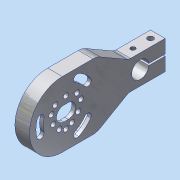
# Autodesk Inventor part: MotorMountingPlate
Saved by Autodesk Inventor 2015 SP1 (Build 190203100, 203)
## iProperties
Created: 2015-06-16
Part Number: MotorMountingPlate
Material: Aluminum 6061
Document SubType Name: Modeling
Designer: YOUR_NAME_HERE
Density: 2.7 g/cm^3
Appearance: Aluminum - Flat
Mass: 93.3221 g
Surface Area: 173.371 cm^2
Volume: 34.5637 cm^3
Author: YOUR_NAME_HERE
Autodesk Inventor part; units mm, degrees
ref_plane "YZ Plane" through (0, 0, 0) normal (1, 0, 0) x (0, 1, 0)
ref_plane "XZ Plane" through (0, 0, 0) normal (0, 1, 0) x (-1, 0, 0)
ref_plane "XY Plane" through (0, 0, 0) normal (0, 0, 1) x (1, 0, 0)
sketch "Sketch1" plane through (0, 0, 0) normal (1, 0, 0) x (0, 1, 0)
  circle A0 centre (0, 0) radius 31.85 construction
  circle A1 centre (0, 64.66) radius 12.75 construction
  line L0 (-44.59, 0) -> (44.59, 0) projected
  line L1 (0, -57.502) -> (0, 122.062) projected
  line L2 (28.575, 96.41) -> (-28.575, 96.41)
  line L3 (-28.575, 96.41) -> (-28.575, -21.59)
  line L4 (-28.575, -21.59) -> (28.575, -21.59)
  line L5 (28.575, -21.59) -> (28.575, 96.41)
  circle A2 centre (0, 64.66) radius 6.35
  circle A3 centre (0, 0) radius 7.5
  dimension "d0" = 63.7
  dimension "d1" = 25.5
  dimension "CC" = 64.66
  dimension "d3" = 21.59
  dimension "d4" = 28.575
  dimension "d5" = 31.75
  dimension "d6" = 15
  dimension "d7" = 12.7
  constraints: 8 end point, 4 centre point, 2 coincident, 2 parallel, 1 horizontal, 1 perpendicular, 1 point on line, 1 other
  measures "d0" diameter of A0
  measures "d1" diameter of A1
  measures "CC" distance of A0.centre A1.centre
  measures "d3" distance from line of L4 A0.centre
  measures "d4" distance from line of L5 A0.centre
  measures "d5" distance from line of A1.centre L2
  measures "d6" diameter of A3
  measures "d7" diameter of A2
extrude "Extrusion1" add sketch "Sketch1" along normal blind 12.7 contours L3 L2 L1 A2 A3 L0 | L0 A3 L1 L4 L3 | L1 A2 L2 L5 L0 A3 | A3 L0 L5 L4 L1
sketch "Sketch2" plane through (12.7, 0, 0) normal (1, 0, 0) x (0, 0, -1)
  circle A0 centre (-64.66, 0) radius 6.35 projected
  circle A1 centre (-64.66, 0) radius 12.5 construction
  circle A2 centre (-64.66, 12.5) radius 2.25
  circle A3 centre (-64.66, -12.5) radius 2.25
  point P0 (0, 0)
  dimension "bolt_circle" = 25
  dimension "d11" = 4.5
  constraints: 3 centre point, 2 point on circle, 2 vertical alignment, 1 coincident, 1 equal radius
  measures "bolt_circle" diameter of A1
  measures "d11" diameter of A2
extrude "Extrusion2" cut sketch "Sketch2" against normal through all contours A2 | A3
sketch "Sketch11" plane through (12.7, 0, 0) normal (1, 0, 0) x (0, 0, -1)
  line L0 (-120.01, 0) -> (45.19, 0)
  line L1 (0, -40.005) -> (0, 40.005)
  circle A0 centre (-64.66, 0) radius 6.35
  circle A1 centre (-64.66, 12.5) radius 2.25
  circle A2 centre (-64.66, -12.5) radius 2.25
  circle A3 centre (-64.66, 0) radius 6.35
  circle A4 centre (-65.66, 0) radius 6.35
  circle A5 centre (-65.66, 0) radius 12.5 construction
  circle A6 centre (-77.295102, 4.568851) radius 2.25
  circle A7 centre (-54.024898, -4.568851) radius 2.25
  line L2 (-77.295102, 4.568851) -> (-54.024898, -4.568851)
  circle A8 centre (-66.66, 0) radius 6.35
  circle A9 centre (-66.66, 0) radius 12.5 construction
  circle A10 centre (-59.430659, -10.197384) radius 2.25
  circle A11 centre (-73.889341, 10.197384) radius 2.25
  line L3 (-59.430659, -10.197384) -> (-73.889341, 10.197384)
  circle A12 centre (-63.66, 0) radius 6.35
  circle A13 centre (-62.66, 0) radius 6.35
  circle A14 centre (-63.66, 0) radius 12.5 construction
  circle A15 centre (-62.66, 0) radius 12.5 construction
  circle A16 centre (-75.660667, -3.497712) radius 2.25
  circle A17 centre (-70.377411, -9.833187) radius 2.25
  circle A18 centre (-54.942589, 9.833187) radius 2.25
  circle A19 centre (-51.659333, 3.497712) radius 2.25
  line L4 (-51.659333, 3.497712) -> (-75.660667, -3.497712)
  line L5 (-70.377411, -9.833187) -> (-54.942589, 9.833187)
  line L6 (-66.66, -6.35) -> (-62.66, -6.35)
  line L7 (-66.66, 6.35) -> (-62.66, 6.35)
  point P0 (0, 0)
  dimension "d62" = 1
  dimension "d67" = 25
  dimension "d84" = 1
  constraints: 17 centre point, 12 end point, 12 equal radius, 12 point on circle, 5 coincident, 4 horizontal, 4 midpoint, 2 tangent, 8 other
  measures "d62" distance of A3.centre A4.centre
  measures "d67" diameter of A5
  measures "d84" distance of A3.centre A12.centre
sketch "Sketch11 outline for Extrusion10" plane through (12.7, 0, 0) normal (1, 0, 0) x (0, 0, -1)
  circle A0 centre (-77.295102, 4.568851) radius 2.25
  circle A1 centre (-54.024898, -4.568851) radius 2.25
  circle A2 centre (-59.430659, -10.197384) radius 2.25
  circle A3 centre (-73.889341, 10.197384) radius 2.25
  circle A4 centre (-75.660667, -3.497712) radius 2.25
  circle A5 centre (-70.377411, -9.833187) radius 2.25
  circle A6 centre (-54.942589, 9.833187) radius 2.25
  circle A7 centre (-51.659333, 3.497712) radius 2.25
  line L0 (-62.66, 6.35) -> (-66.66, 6.35)
  arc A8 (-66.66, 6.35) -> (-66.66, -6.35) centre (-66.66, 0) ccw
  line L1 (-66.66, -6.35) -> (-62.66, -6.35)
  arc A9 (-62.66, -6.35) -> (-62.66, 6.35) centre (-62.66, 0) ccw
extrude "Extrusion10" cut sketch "Sketch11 outline for Extrusion10" against normal through all
sketch "Sketch4" plane through (0, 0, 0) normal (-1, 0, 0) x (0, 0, 1)
  line L0 (66.66, -6.35) -> (62.66, -6.35)
  arc A0 (62.66, 6.35) -> (62.66, -6.35) centre (62.66, 0) ccw
  line L1 (62.66, 6.35) -> (66.66, 6.35)
  arc A1 (66.66, -6.35) -> (66.66, 6.35) centre (66.66, 0) ccw
  circle A2 centre (51.659333, 3.497712) radius 2.25
  circle A3 centre (70.377411, -9.833187) radius 2.25
  circle A4 centre (73.889341, 10.197384) radius 2.25
  circle A5 centre (54.024898, -4.568851) radius 2.25
  circle A6 centre (77.295102, 4.568851) radius 2.25
  circle A7 centre (59.430659, -10.197384) radius 2.25
  circle A8 centre (75.660667, -3.497712) radius 2.25
  circle A9 centre (54.942589, 9.833187) radius 2.25
  circle A10 centre (64.66, 12.5) radius 2.25
  circle A11 centre (64.66, -12.5) radius 2.25
  circle A12 centre (0, 0) radius 7.5
  line L2 (96.41, 28.575) -> (96.41, -28.575)
  line L3 (-21.59, 28.575) -> (96.41, 28.575)
  line L4 (-21.59, -28.575) -> (-21.59, 28.575)
  line L5 (96.41, -28.575) -> (-21.59, -28.575)
  line L6 (62.66, 0) -> (66.66, 0) construction
  line L7 (62.66, -26) -> (66.66, -26)
  line L8 (66.66, 26) -> (62.66, 26)
  arc A13 (62.66, 26) -> (62.66, -26) centre (62.66, 0) ccw
  arc A14 (66.66, -26) -> (66.66, 26) centre (66.66, 0) ccw
  point P0 (64.66, 0)
  dimension "d116" = 52
  constraints: 8 end point, 4 point on circle, 4 tangent, 2 centre point, 1 horizontal, 1 midpoint, 1 parallel
  measures "d116" distance between parallel lines of L7 L8
extrude "Extrusion4" cut sketch "Sketch4" against normal blind 9.525 contours A13 L8 A14 L7
sketch "Sketch6" plane through (0, 0, 0) normal (-1, 0, 0) x (0, 0, 1)
  line L0 (-45.19, 0) -> (120.01, 0)
  line L1 (-21.59, -28.575) -> (-21.59, 28.575)
  line L2 (-21.59, 28.575) -> (96.41, 28.575)
  line L3 (96.41, 28.575) -> (96.41, -28.575)
  line L4 (96.41, -28.575) -> (-21.59, -28.575)
  line L5 (-21.59, -0.79375) -> (-7.457879, -0.79375)
  line L6 (-7.457879, 0.79375) -> (-21.59, 0.79375)
  circle A0 centre (0, 0) radius 7.5
  line L7 (-21.59, 0.79375) -> (-21.59, -0.79375)
  point P0 (-7.5, 0)
  dimension "d30" = 1.5875
  constraints: 6 end point, 3 point on circle, 2 point on line, 1 collinear, 1 horizontal, 1 parallel, 1 other
  measures "d30" distance between parallel lines of L5 L6
extrude "Extrusion5" cut sketch "Sketch6" against normal through all contours L1 L6 A0 L0 | L0 A0 L5 L1
sketch "Sketch7" plane through (0, 0, 0) normal (-1, 0, 0) x (0, 0, 1)
  arc A0 (-7.457879, -0.79375) -> (-7.457879, 0.79375) centre (0, 0) ccw
  line L0 (-21.59, 0.79375) -> (-7.457879, 0.79375)
  line L1 (-7.457879, -0.79375) -> (-21.59, -0.79375)
  line L2 (-21.59, 0.79375) -> (-21.59, 28.575)
  line L3 (-21.59, -28.575) -> (-21.59, -0.79375)
  line L4 (96.41, -28.575) -> (-21.59, -28.575)
  line L5 (-21.59, 28.575) -> (96.41, 28.575)
  line L6 (-21.59, 12.58) -> (10.16, 12.58)
  line L7 (10.16, 12.58) -> (37.864153, 28.575)
  line L8 (-21.59, -12.58) -> (10.16, -12.58)
  line L9 (10.16, -12.58) -> (37.864153, -28.575)
  line L10 (-45.19, 0) -> (120.01, 0)
  point P0 (0, 7.5)
  dimension "d34" = 31.75
  dimension "d118" = 30
  dimension "d119" = 30
  dimension "d124" = 5.08
  constraints: 8 end point, 4 point on line, 2 horizontal, 2 vertical alignment, 1 point on circle, 1 other
  measures "d34" distance of L6.start L6.end
  measures "d118" angle of L5 L7
  measures "d119" angle of L4 L9
  measures "d124" distance from line of L6 point (0, 7.5)
extrude "Extrusion6" cut sketch "Sketch7" against normal through all
sketch "Sketch10" plane through (0, 0, 0) normal (-1, 0, 0) x (0, 0, 1)
  line L0 (10.16, 12.58) -> (-21.59, 12.58)
  line L1 (-21.59, 0.79375) -> (-21.59, 12.58)
  line L2 (-21.59, 0.79375) -> (-7.457879, 0.79375)
  arc A0 (-7.457879, -0.79375) -> (-7.457879, 0.79375) centre (0, 0) ccw
  line L3 (-7.457879, -0.79375) -> (-21.59, -0.79375)
  line L4 (-21.59, -12.58) -> (-21.59, -0.79375)
  line L5 (-21.59, -12.58) -> (10.16, -12.58)
  line L6 (10.16, -12.58) -> (37.864153, -28.575)
  line L7 (96.41, -28.575) -> (37.864153, -28.575)
  line L8 (96.41, 28.575) -> (96.41, -28.575)
  line L9 (37.864153, 28.575) -> (96.41, 28.575)
  line L10 (37.864153, 28.575) -> (10.16, 12.58)
  line L11 (-45.19, 0) -> (120.01, 0)
  arc A1 (17.859227, -9.692802) -> (17.859227, 9.692802) centre (0, 0) ccw
  arc A2 (62.66, 26) -> (62.66, -26) centre (62.66, 0) ccw construction
  line L12 (62.66, 26) -> (66.66, 26)
  line L13 (66.66, -26) -> (62.66, -26)
  line L14 (17.859227, 9.692802) -> (46.104122, 26)
  line L15 (17.859227, -9.692802) -> (46.104122, -26)
  line L16 (37.864153, 28.575) -> (10.16, 12.58)
  line L17 (46.104122, 26) -> (62.66, 26)
  line L18 (46.104122, -26) -> (62.66, -26)
  line L19 (62.66, 26) -> (66.66, 26)
  line L20 (62.66, -26) -> (66.66, -26)
  arc A3 (66.66, -26) -> (66.66, 26) centre (66.7, 0) ccw
  dimension "d103" = 20.32
  dimension "d120" = 6.35
  constraints: 12 end point, 4 point on circle, 2 centre point, 2 coincident, 2 parallel, 2 vertical alignment, 1 collinear, 1 horizontal, 1 point on line, 1 tangent
  measures "d103" radius of A1
  measures "d120" distance between parallel lines of L10 L14
extrude "Extrusion8" cut sketch "Sketch10" against normal blind 9.525 contours A3 L13 L18 L15 A1 L11 | L11 A1 L14 L17 L12 A3
sketch "Sketch8" plane through (0, 12.58, 10.16) normal (0, 1, 0) x (1, 0, 0)
  line L0 (12.7, 17.617879) -> (12.7, 17.617879)
  circle A0 centre (6.35, 25.4) radius 2.5527
  line L1 (0, 31.75) -> (12.7, 31.75)
  line L2 (0, 17.617879) -> (0, 17.617879)
  line L3 (12.7, 17.617879) -> (0, 17.617879)
  line L4 (0, 17.617879) -> (12.7, 17.617879)
  point P0 (0, 10.16)
  point P1 (6.35, 31.75)
  dimension "d38" = 6.35
  dimension "d39" = 5.1054
  constraints: 1 centre point, 1 midpoint, 1 vertical alignment
  measures "d38" distance from line of L1 A0.centre
  measures "d39" diameter of A0
extrude "Extrusion7" cut sketch "Sketch8" against normal through all
fillet "Fillet5" radius 28.575 2 edges at (6.35, 28.575, 96.41) (6.35, -28.575, 96.41)
fillet "Fillet5" radius 12.7 2 edges at (6.35, 28.575, 37.8642) (6.35, -28.575, 37.8642)
fillet "Fillet5" radius 6.35 2 edges at (6.35, 12.58, 10.16) (6.35, -12.58, 10.16)
fillet "Fillet6" radius 6.35 6 edges at (4.7625, 26, 46.1041) (4.7625, -26, 46.1041) (4.7625, -26, 66.66) (4.7625, 26, 66.66) (4.7625, 9.6928, 17.8592) (4.7625, -9.6928, 17.8592)
sketch "Sketch12" plane through (9.525, 0, 0) normal (-1, 0, 0) x (0, 0, 1)
  arc A0 (86.863737, -5.949473) -> (86.863737, 5.949473) centre (64.66, 0) ccw construction
  arc A1 (89.930551, -6.771224) -> (89.930551, 6.771224) centre (64.66, 0) ccw
  arc A2 (83.796922, -5.127723) -> (83.796922, 5.127723) centre (64.66, 0) ccw
  arc A3 (83.796922, -5.127723) -> (89.930551, -6.771224) centre (86.863737, -5.949473) ccw
  arc A4 (89.930551, 6.771224) -> (83.796922, 5.127723) centre (86.863737, 5.949473) ccw
  line L0 (86.863737, -5.949473) -> (64.66, 0) construction
  line L1 (64.66, 0) -> (86.863737, 5.949473) construction
  line L2 (-45.19, 0) -> (120.01, 0)
  arc A5 (54.945274, 20.833297) -> (45.830152, 13.184802) centre (64.66, 0) ccw construction
  arc A6 (53.603461, 23.710824) -> (43.229344, 15.005907) centre (64.66, 0) ccw
  arc A7 (56.287087, 17.95577) -> (48.43096, 11.363696) centre (64.66, 0) ccw
  arc A8 (56.287087, 17.95577) -> (53.603461, 23.710824) centre (54.945274, 20.833297) ccw
  arc A9 (43.229344, 15.005907) -> (48.43096, 11.363696) centre (45.830152, 13.184802) ccw
  line L3 (54.945274, 20.833297) -> (64.66, 0) construction
  line L4 (64.66, 0) -> (45.830152, 13.184802) construction
  circle A10 centre (64.66, 0) radius 6.35
  arc A11 (43.229344, -15.005907) -> (53.603461, -23.710824) centre (64.66, 0) ccw
  arc A12 (48.43096, -11.363696) -> (56.287087, -17.95577) centre (64.66, 0) ccw
  arc A13 (53.603461, -23.710824) -> (56.287087, -17.95577) centre (54.945274, -20.833297) ccw
  arc A14 (48.43096, -11.363696) -> (43.229344, -15.005907) centre (45.830152, -13.184802) ccw
  point P0 (0, 0)
  dimension "d106" = 19.812
  dimension "d107" = 6.35
  dimension "d108" = 30
  dimension "d111" = 19.812
  dimension "d112" = 6.35
  dimension "d113" = 30
  dimension "d122" = 100
  constraints: 28 point on circle, 14 centre point, 8 end point, 8 tangent, 7 symmetric about line, 2 coincident, 4 other
  measures "d106" radius of A2
  measures "d107" radial gap between concentric circles of A1 A2
  measures "d108" angle of L0 L1
  measures "d111" radius of A7
  measures "d112" radial gap between concentric circles of A6 A7
  measures "d113" angle of L3 L4
  measures "d122" angle of L1 L3
extrude "Extrusion11" cut sketch "Sketch12" against normal through all
sketch "Sketch13" plane through (0, 12.58, -21.59) normal (0, 1, 0) x (1, 0, 0)
  circle A0 centre (6.35, -21.59) radius 2.0193
  line L0 (0, 0) -> (12.7, 0) projected
  point P0 (0, -21.59)
  point P1 (6.35, 0)
  dimension "d125" = 4.0386
  dimension "d128" = 21.59
  constraints: 1 centre point, 1 midpoint, 1 vertical alignment
  measures "d125" diameter of A0
  measures "d128" distance from line of L0 A0.centre
extrude "Extrusion12" cut sketch "Sketch13" against normal up to surface (12.58 mm away)
thread "Thread3" size "10-32 UNF" class "2B" standard "ANSI Unified Screw Threads" full length
equation "\"d67\" = bolt_circle"
body "Solid1"
